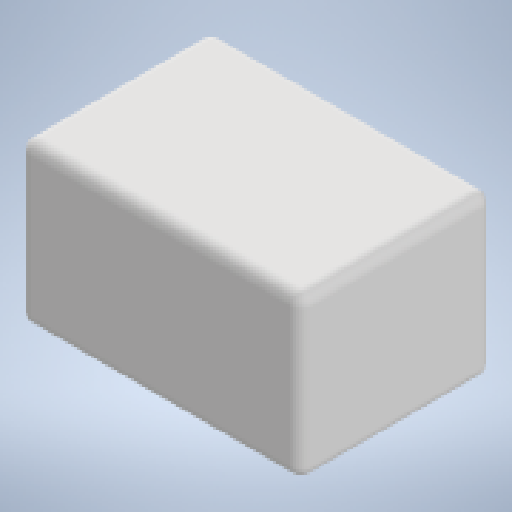
# Autodesk Inventor part: 电池
Saved by Autodesk Inventor 2025.1 (Build 291241000, 241)
## iProperties
Created: 2025-09-03
Part Number: 电池
Material: 常规
Document SubType Name: Modeling
Designer: Piw
Density: 1 g/cm^3
Appearance: 默认
Author: Piw
Autodesk Inventor part; units mm, degrees
ref_plane "YZ Plane" through (0, 0, 0) normal (1, 0, 0) x (0, 1, 0)
ref_plane "XZ Plane" through (0, 0, 0) normal (0, 1, 0) x (-1, 0, 0)
ref_plane "XY Plane" through (0, 0, 0) normal (0, 0, 1) x (1, 0, 0)
sketch "草图1" plane through (0, 0, 0) normal (1, 0, 0) x (0, 1, 0)
  line L0 (0, 0) -> (-56, 0)
  line L1 (-56, 0) -> (-56, -67)
  line L2 (-56, -67) -> (0, -67)
  line L3 (0, -67) -> (0, 0)
  dimension "d0" = 67
  dimension "d1" = 56
  constraints: 8 end point, 2 parallel, 1 horizontal, 1 perpendicular
  measures "d0" distance of L2.end L0.start
  measures "d1" distance of L1.end L2.end
extrude "拉伸1" add sketch "草图1" along normal blind 98.5
fillet "圆角1" radius 4 12 edges at (98.5, 0, -33.5) (98.5, -28, -67) (98.5, -28, 0) (98.5, -56, -33.5) (49.25, 0, 0) (49.25, 0, -67) (49.25, -56, 0) (49.25, -56, -67) (0, 0, -33.5) (0, -28, 0) (0, -28, -67) (0, -56, -33.5)
